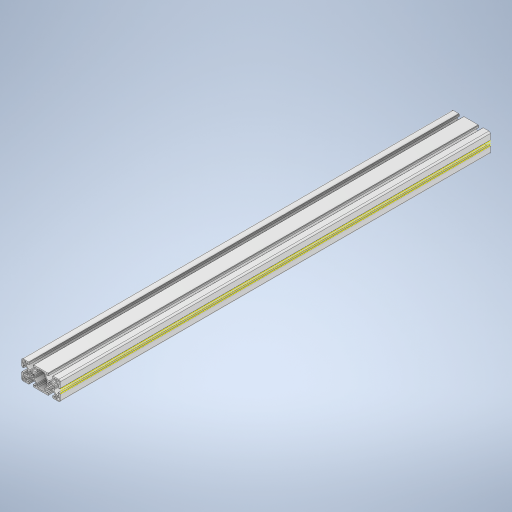
# Autodesk Inventor part: Alu_Profile_40x80x300-01
Saved by Autodesk Inventor 2023 (Build 270158000, 158)
## iProperties
Category: Profiles
Company: CMBSolutions
Created: 2022-05-12
Part Number: Alu_Profile_40x80x300-01
Material: Aluminum 6061 T6 0 Cold Formed
Document SubType Name: Modeling
Designer: Maurice
Density: 2.7 g/cm^3
Appearance: Satin
User Status: Completed
Catalog Web Link: https://www.vallder.com/en/c/alu-profile/alu-profile-40x80-detail
Description: These structural aluminum profiles are extruded from a AI6060-T5 material.
Vendor: Vallder
Stock Number: 1115000
Mass: 818.498 g
Surface Area: 2502.86 cm^2
Volume: 303.147 cm^3
length: 890.000 mm
PriceNoTax: € 0,03 per mm
Author: Maurice
Title: Alu Profile 40x80x300
Subject: Extruded profiles
Autodesk Inventor part; units mm, degrees
ref_plane "YZ Plane" through (0, 0, 0) normal (1, 0, 0) x (0, 1, 0)
ref_plane "XZ Plane" through (0, 0, 0) normal (0, 1, 0) x (-1, 0, 0)
ref_plane "XY Plane" through (0, 0, 0) normal (0, 0, 1) x (1, 0, 0)
sketch "Sketch1" plane through (0, 0, 0) normal (0, 0, 1) x (1, 0, 0)
  line L0 (0, 0) -> (-12.9793, 0) construction
  line L1 (-40, 5.3) -> (-40, 17)
  line L2 (-37, 20) -> (-25.3, 20)
  line L3 (0, 20) -> (0, 17.6)
  arc A0 (-37, 20) -> (-40, 17) centre (-37, 17) ccw
  arc A1 (0, 17.6) -> (-6.38, 16.6546) centre (0, -4.4) ccw
  line L4 (-14.7, 20) -> (-14.7, 19)
  line L5 (-14.7, 19) -> (-15.9, 19)
  line L6 (-15.9, 19) -> (-15.9, 15.7)
  line L7 (-15.9, 15.7) -> (-13, 15.7)
  line L8 (-12, 17) -> (-12, 17)
  line L9 (-10, 15) -> (-10, 11.56)
  line L10 (-17.3, 7.7) -> (-19.3, 7.7)
  line L11 (-19.3, 7.7) -> (-20, 7)
  line L12 (-20, 7) -> (-20, 20) construction
  arc A2 (-4.0452, 15.7) -> (-6.38, 16.6546) centre (-5.8, 14.7405) ccw construction
  arc A3 (-6.38, 16.6546) -> (-7.8, 14.7405) centre (-5.8, 14.7405) ccw
  line L13 (-10, 11.56) -> (-12.6836, 8.8721) construction
  line L14 (-12.6836, 8.8721) -> (-14.6269, 6.8843) construction
  line L15 (-14.6269, 6.8843) -> (-16.3882, 6.8895) construction
  line L16 (-16.3882, 6.8895) -> (-16.3882, 7.35) construction
  line L17 (-16.3882, 7.35) -> (-16.8508, 7.7) construction
  line L18 (-16.8508, 7.7) -> (-17.3, 7.7) construction
  spline S0 degree 4 poles (-10, 11.56) (-12.6836, 8.8721) (-14.6269, 6.8843) (-16.3882, 6.8895) (-16.3882, 7.35) (-16.8508, 7.7) (-17.3, 7.7) knots 1 1 1 1 1 2 3 4 4 4 4 4
  arc A4 (-13, 15.7) -> (-12.6, 16.1) centre (-13, 16.1) ccw
  arc A5 (-10, 15) -> (-12, 17) centre (-12, 15) ccw
  line L19 (-7.8, 14.7405) -> (-7.8, 11.92)
  arc A6 (-8.44, 10) -> (-7.8, 11.92) centre (-11, 11.92) ccw
  line L20 (-20, 0) -> (-8.6828, 11.3172) construction
  line L21 (-12.3, 2.7) -> (-12.3, 0.7)
  line L22 (-12.3, 0.7) -> (-12.9793, 0)
  line L23 (-8.44, 10) -> (-11.1279, 7.3164) construction
  line L24 (-11.1279, 7.3164) -> (-13.1157, 5.3731) construction
  line L25 (-13.1157, 5.3731) -> (-13.1105, 3.6118) construction
  line L26 (-13.1105, 3.6118) -> (-12.65, 3.6118) construction
  line L27 (-12.65, 3.6118) -> (-12.3, 3.1492) construction
  line L28 (-12.3, 3.1492) -> (-12.3, 2.7) construction
  spline S1 degree 4 poles (-8.44, 10) (-11.1279, 7.3164) (-13.1157, 5.3731) (-13.1105, 3.6118) (-12.65, 3.6118) (-12.3, 3.1492) (-12.3, 2.7) knots 1 1 1 1 1 2 3 4 4 4 4 4
  line L29 (0, 17.6) -> (0, 0) construction
  line L30 (-12.9793, 0) -> (-40, 0)
  line L31 (-25.3, 20) -> (-25.3, 19)
  line L32 (-25.3, 19) -> (-24.1, 19)
  line L33 (-24.1, 19) -> (-24.1, 15.7)
  line L34 (-30, 15) -> (-30, 11.56)
  line L35 (-22.7, 7.7) -> (-20.7, 7.7)
  line L36 (-20.7, 7.7) -> (-20, 7)
  line L37 (-30, 11.56) -> (-27.3164, 8.8721) construction
  line L38 (-27.3164, 8.8721) -> (-25.3731, 6.8843) construction
  line L39 (-25.3731, 6.8843) -> (-23.6118, 6.8895) construction
  line L40 (-23.6118, 6.8895) -> (-23.6118, 7.35) construction
  line L41 (-23.6118, 7.35) -> (-23.1492, 7.7) construction
  line L42 (-23.1492, 7.7) -> (-22.7, 7.7) construction
  spline S2 degree 4 poles (-30, 11.56) (-27.3164, 8.8721) (-25.3731, 6.8843) (-23.6118, 6.8895) (-23.6118, 7.35) (-23.1492, 7.7) (-22.7, 7.7) knots 1 1 1 1 1 2 3 4 4 4 4 4
  arc A7 (-27.4, 16.1) -> (-27, 15.7) centre (-27, 16.1) ccw
  arc A8 (-28, 17) -> (-30, 15) centre (-28, 15) ccw
  line L43 (-27, 15.7) -> (-24.1, 15.7)
  line L44 (-25.3, 20) -> (-14.7, 20) construction
  line L45 (-14.7, 20) -> (0, 20)
  line L46 (-20, 0) -> (-40, 20) construction
  line L47 (-40, 5.3) -> (-39, 5.3)
  line L48 (-39, 5.3) -> (-39, 4.1)
  line L49 (-39, 4.1) -> (-35.7, 4.1)
  arc A9 (-35.7, 7) -> (-36.1, 7.4) centre (-36.1, 7) ccw
  arc A10 (-35, 10) -> (-37, 8) centre (-35, 8) ccw
  line L50 (-35, 10) -> (-31.56, 10)
  spline S3 degree 4 poles (-31.56, 10) (-28.8721, 7.3164) (-26.8843, 5.3731) (-26.8895, 3.6118) (-27.35, 3.6118) (-27.7, 3.1492) (-27.7, 2.7) knots 1 1 1 1 1 2 3 4 4 4 4 4
  line L51 (-27.7, 2.7) -> (-27.7, 0.7)
  line L52 (-27.7, 0.7) -> (-27, 0)
  line L53 (-31.56, 10) -> (-28.8721, 7.3164) construction
  line L54 (-28.8721, 7.3164) -> (-26.8843, 5.3731) construction
  line L55 (-26.8843, 5.3731) -> (-26.8895, 3.6118) construction
  line L56 (-26.8895, 3.6118) -> (-27.35, 3.6118) construction
  line L57 (-27.35, 3.6118) -> (-27.7, 3.1492) construction
  line L58 (-27.7, 3.1492) -> (-27.7, 2.7) construction
  line L59 (-35.7, 7) -> (-35.7, 4.1)
  arc A11 (-15, 0) -> (-15.1277, 1.1229) centre (-20, 0) ccw
  arc A12 (-14, 0) -> (-14.1534, 1.3479) centre (-20, 0) ccw construction
  line L60 (-20, 0) -> (-14.4567, 2.2961) construction
  line L61 (-20, 0) -> (-14, 0) construction
  line L62 (-14.9212, 3.1946) -> (-15.7692, 2.6647)
  line L63 (-14.1534, 1.3479) -> (-15.1277, 1.1229)
  arc A13 (-15.7692, 2.6647) -> (-16.4645, 3.5355) centre (-20, 0) ccw
  arc A14 (-15.1277, 1.1229) -> (-15.7692, 2.6647) centre (-20, 0) ccw construction
  line L64 (-15, 0) -> (-12.9793, 0)
  arc A15 (-14.1534, 1.3479) -> (-14.9212, 3.1946) centre (-20, 0) ccw
  arc A16 (-14.9212, 3.1946) -> (-15.7574, 4.2426) centre (-20, 0) ccw construction
  arc A17 (-16.4645, 3.5355) -> (-17.3488, 4.2392) centre (-20, 0) ccw
  line L65 (-16.8189, 5.0873) -> (-17.3488, 4.2392)
  arc A18 (-16.8189, 5.0873) -> (-18.6677, 5.8502) centre (-20, 0) ccw
  line L66 (-18.6677, 5.8502) -> (-18.8926, 4.8758)
  arc A19 (-18.8926, 4.8758) -> (-20, 5) centre (-20, 0) ccw
  arc A20 (-20, 5) -> (-21.1229, 4.8723) centre (-20, 0) ccw
  line L67 (-21.3479, 5.8466) -> (-21.1229, 4.8723)
  arc A21 (-21.3479, 5.8466) -> (-23.1946, 5.0788) centre (-20, 0) ccw
  line L68 (-23.1946, 5.0788) -> (-22.6647, 4.2308)
  arc A22 (-22.6647, 4.2308) -> (-23.5355, 3.5355) centre (-20, 0) ccw
  arc A23 (-23.5355, 3.5355) -> (-24.2392, 2.6512) centre (-20, 0) ccw
  line L69 (-25.0873, 3.1811) -> (-24.2392, 2.6512)
  arc A24 (-25.0873, 3.1811) -> (-25.8502, 1.3323) centre (-20, 0) ccw
  line L70 (-25.8502, 1.3323) -> (-24.8758, 1.1074)
  arc A25 (-24.8758, 1.1074) -> (-25, 0) centre (-20, 0) ccw
  line L71 (-25, 0) -> (-27, 0)
  arc A26 (-37, 8) -> (-36.4, 7.4) centre (-36.4, 8) ccw
  arc A27 (-27.4, 16.4) -> (-28, 17) centre (-28, 16.4) ccw
  arc A28 (-12, 17) -> (-12.6, 16.4) centre (-12, 16.4) ccw
  line L72 (-36.4, 7.4) -> (-36.1, 7.4)
  line L73 (-27.4, 16.4) -> (-27.4, 16.1)
  line L74 (-12.6, 16.4) -> (-12.6, 16.1)
  point P0 (-12.6, 15.7)
  point P1 (-14.1534, 1.3479)
  point P2 (-25, 0)
  dimension "d0" = 40
  dimension "d1" = 20
  dimension "d4" = 3
  dimension "d17" = 2.4
  dimension "d18" = 22
  dimension "d19" = 5.3
  dimension "d20" = 20
  dimension "d21" = 4.1
  dimension "d22" = 3.3
  dimension "d23" = 1
  dimension "d24" = 3.3
  dimension "d25" = 8
  dimension "d26" = 0.7
  dimension "d27" = 2.7
  dimension "d28" = 4.14
  dimension "d29" = 3
  dimension "d30" = 10
  dimension "d31" = 0.7
  dimension "d32" = 2
  dimension "d33" = 4.2
  dimension "d34" = 7.8
  dimension "d36" = 0.4
  dimension "d38" = 2
  dimension "d40" = 3.2
  dimension "d41" = 2.2
  dimension "d42" = 1.1
  dimension "d43" = 45
  dimension "d44" = 5
  dimension "d45" = 6
  dimension "d46" = 22.5
  dimension "d47" = 19
  dimension "d48" = 2
  dimension "d49" = 13
  constraints: 110 end point, 65 point on circle, 47 symmetric about line, 29 centre point, 14 point on line, 11 perpendicular, 9 parallel, 8 tangent, 5 coincident, 5 horizontal, 4 vertical, 2 collinear, 2 vertical alignment, 1 equal length, 1 midpoint, 16 other
  measures "d0" distance of L46.end L3.start
  measures "d1" distance of L30.end L46.end
  measures "d4" radius of A0
  measures "d17" distance of L3.start L3.end
  measures "d18" radius of A1
  measures "d19" distance between parallel lines of L4 L12
  measures "d20" distance from line of L0.start L12
  measures "d21" distance between parallel lines of L6 L12
  measures "d22" distance of L5.end L6.end
  measures "d23" distance of L4.start L4.end
  measures "d24" distance of L6.end point (-12.6, 15.7)
  measures "d25" distance between parallel lines of L10 L7
  measures "d26" horizontal distance of L11.end L10.end
  measures "d27" distance from line of L12 L10.start
  measures "d28" distance from line of L9.end L7
  measures "d29" distance between parallel lines of L2 L8
  measures "d30" distance between parallel lines of L12 L9
  measures "d31" horizontal distance of L11.end L10.end
  measures "d32" radius of A2
  measures "d33" distance from line of L9 A2.centre
  measures "d34" horizontal distance of L0.start L19.start
  measures "d36" radius of A4
  measures "d38" radius of A5
  measures "d40" radius of A6
  measures "d41" distance of L13.end L23.end
  measures "d42" distance from line of L20 L13.end
  measures "d43" angle of L0 L20
  measures "d44" radius of A11
  measures "d45" radius of A12
  measures "d46" angle of L61 L60
  measures "d47" angle of L63 L62
  measures "d48" distance of L63.start L62.start
  measures "d49" angle of L30 L63
extrude "Extrusion1" add sketch "Sketch1" along normal blind 890 contours L1 A0 L2 L31 L32 L33 L43 A7 L73 A27 A8 L34 S2 L35 L36 L11 L10 S0 L9 A5 A28 L74 A4 L7 L6 L5 L4 L45 L3 A1 A3 L19 A6 S1 L21 L22 L30 A11 L63 A15 L62 A13 A17 L65 A18 L66 A19 A20 L67 A21 L68 A22 A23 L69 A24 L70 A25 L52 L51 S3 L50 A10 A26 L72 A9 L59 L49 L48 L47
sketch "Sketch3" plane through (0, 0, 890) normal (0, 0, 1) x (1, 0, 0)
  line L0 (-40, 17) -> (-40, 5.3) projected
  arc A0 (-37, 20) -> (-40, 17) centre (-37, 17) ccw projected
  line L1 (-25.3, 20) -> (-37, 20) projected
  line L2 (-30, 11.56) -> (-30, 15) projected
  line L3 (-35, 10) -> (-31.56, 10) projected
  line L4 (-38.1, 11.03) -> (-38.1, 11.53) construction
  arc A1 (-37, 18.1) -> (-38.1, 17) centre (-37, 17) ccw
  line L5 (-37, 18.1) -> (-31.53, 18.1)
  line L6 (-31.9, 12.4) -> (-31.9, 15)
  line L7 (-35, 11.9) -> (-32.4, 11.9)
  arc A2 (-32.4, 11.9) -> (-31.9, 12.4) centre (-32.4, 12.4) ccw
  arc A3 (-38.1, 11.53) -> (-37.275, 11.15) centre (-37.6, 11.53) ccw
  arc A4 (-35, 11.9) -> (-37.275, 11.15) centre (-35, 8.0745) ccw
  arc A5 (-37.275, 11.15) -> (-38.1, 11.53) centre (-37.6, 11.53) ccw construction
  line L8 (-38.1, 11.53) -> (-38.1, 17)
  arc A6 (-31.15, 17.275) -> (-31.53, 18.1) centre (-31.53, 17.6) ccw
  arc A7 (-31.15, 17.275) -> (-31.9, 15) centre (-28.0745, 15) ccw
  arc A8 (-31.53, 18.1) -> (-31.15, 17.275) centre (-31.53, 17.6) ccw construction
  line L9 (-31.53, 18.1) -> (-31.03, 18.1) construction
  point P0 (0, 0)
  dimension "d56" = 1.9
  dimension "d57" = 5.97
  dimension "d58" = 5.97
  dimension "d59" = 1.9
  dimension "d60" = 1.9
  dimension "d61" = 0.5
  dimension "d63" = 1
  dimension "d64" = 0.5
  dimension "d65" = 1
  dimension "d66" = 0.5
  constraints: 16 point on circle, 12 end point, 8 centre point, 8 tangent, 2 parallel
  measures "d56" distance between parallel lines of L0 L4
  measures "d57" distance of L5.start L9.end
  measures "d58" distance of L4.start L8.end
  measures "d59" distance between parallel lines of L2 L6
  measures "d60" distance between parallel lines of L3 L7
  measures "d61" radius of A2
  measures "d63" diameter of A3
  measures "d64" horizontal distance of L4.start A3.centre
  measures "d65" diameter of A6
  measures "d66" horizontal distance of L9.end A6.centre
extrude "Extrusion2" cut sketch "Sketch3" against normal through all
mirror "Mirror1" about plane through (-27, 0, 0) normal (0, -1, 0)
mirror "Mirror2" about plane through (0, 17.6, 0) normal (1, 0, 0)
sketch "Sketch4" plane through (40, -5.3, 890) normal (1, 0, 0) x (0, 0, -1)
  line L0 (890, 1.2) -> (0, 1.2) projected
  line L1 (890, 9.4) -> (0, 9.4) projected
  line L2 (890, 5.3) -> (0, 5.3) projected
equation "\"d24\" = d22"
equation "\"d31\" = d26"
body "Solid1"
